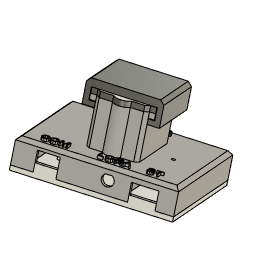
PicoTracker Lora Jig_1.1a v7 (Autodesk Fusion 360 design; units mm, degrees)
Autodesk Fusion 360 part; units mm, degrees
sketch "Sketch1" plane through (0, 0, 0) normal (0, 0, 1) x (1, 0, 0)
  line L0 (-14.5, -3.5) -> (-14.5, 46.5)
  line L1 (-14.5, 46.5) -> (45.5, 46.5)
  line L2 (45.5, 46.5) -> (45.5, -3.5)
  line L3 (-16.5, -5.5) -> (-16.5, 48.5)
  line L4 (-16.5, 48.5) -> (47.5, 48.5)
  line L5 (47.5, 48.5) -> (47.5, -5.5)
  line L6 (-14.5, 46.5) -> (20.5, 46.5)
  line L7 (20.5, 46.5) -> (20.5, 41.5)
  line L8 (20.5, 41.5) -> (-14.5, 41.5)
  line L9 (-14.5, 41.5) -> (-14.5, 46.5)
  line L10 (-14.5, 24.2) -> (20.5, 24.2)
  line L11 (20.5, 24.2) -> (20.5, 21.2)
  line L12 (20.5, 21.2) -> (-14.5, 21.2)
  line L13 (-14.5, 21.2) -> (-14.5, 24.2)
  line L14 (-14.5, 39.5) -> (-16.5, 39.5)
  line L15 (-14.5, 26.2) -> (-16.5, 26.2)
  line L16 (29.5, 46.5) -> (33.5, 46.5)
  line L17 (33.5, 46.5) -> (33.5, 39.5)
  line L18 (33.5, 39.5) -> (29.5, 39.5)
  line L19 (29.5, 39.5) -> (29.5, 46.5)
  line L20 (29.5, 21.2) -> (33.5, 21.2)
  line L21 (33.5, 21.2) -> (33.5, 26.2)
  line L22 (33.5, 26.2) -> (29.5, 26.2)
  line L23 (29.5, 26.2) -> (29.5, 21.2)
  line L24 (20.5, 41.5) -> (20.5, 24.2)
  circle A0 centre (14.5, 32.85) radius 1
  line L25 (-14.5, 1.5) -> (-14.5, -3.5)
  line L26 (45.5, 1.5) -> (45.5, -3.5)
  line L27 (45.5, 46.5) -> (40.5, 46.5)
  line L28 (40.5, 46.5) -> (40.5, 41.5)
  line L29 (40.5, 41.5) -> (45.5, 41.5)
  line L30 (45.5, 41.5) -> (45.5, 46.5)
  circle A1 centre (43, 44) radius 0.9
  circle A2 centre (43, -26) radius 0.9
  circle A3 centre (-12, -26) radius 0.9
  circle A4 centre (-12, 44) radius 0.9
  line L31 (30.5, 0) -> (-1, 0)
  line L32 (-1, 0) -> (-1, 20.5)
  line L33 (-1, 20.5) -> (30.5, 20.5)
  line L34 (30.5, 20.5) -> (30.5, 0)
  arc A5 (-1, 12.75) -> (-1, 7.75) centre (-1, 10.25) ccw
  arc A6 (-1, 15.25) -> (-1, 5.25) centre (-1, 10.25) ccw
  line L35 (-3.5, -2.5) -> (-3.5, 23)
  line L36 (-3.5, 23) -> (33, 23)
  line L37 (33, 23) -> (33, -2.5)
  line L38 (33, -2.5) -> (-3.5, -2.5)
  circle A7 centre (29.1, 10.1) radius 0.85
  circle A8 centre (27.945, 2.48) radius 0.85
  circle A9 centre (25.405, 2.48) radius 0.85
  circle A10 centre (22.865, 2.48) radius 0.85
  circle A11 centre (20.325, 2.48) radius 0.85
  circle A12 centre (17.785, 2.48) radius 0.85
  circle A13 centre (15.245, 2.48) radius 0.85
  circle A14 centre (1.1, 10.1) radius 0.85
  circle A15 centre (1.1, 7.05) radius 0.85
  circle A16 centre (1.1, 13.3) radius 0.85
  circle A17 centre (1.1, 17.1) radius 0.85
  line L39 (26.5, 20.5) -> (3, 20.5)
  line L40 (3, 20.5) -> (3, 4)
  line L41 (26.5, 4) -> (26.5, 20.5)
  line L42 (26.5, 4) -> (3, 4)
  line L43 (14.75, 20.5) -> (14.75, 0)
  circle A18 centre (12.705, 2.48) radius 0.85
  circle A19 centre (10.165, 2.48) radius 0.85
  circle A20 centre (7.625, 2.48) radius 0.85
  circle A21 centre (5.085, 2.48) radius 0.85
  line L44 (-16.5, -5.5) -> (-16.5, -30.5)
  line L45 (-16.5, -30.5) -> (47.5, -30.5)
  line L46 (47.5, -30.5) -> (47.5, -5.5)
  line L47 (-14.5, -7.5) -> (-14.5, -28.5)
  line L48 (-14.5, -28.5) -> (45.5, -28.5)
  line L49 (45.5, -28.5) -> (45.5, -7.5)
  line L50 (45.5, -7.5) -> (45.5, -3.5)
  line L51 (-14.5, -7.5) -> (-14.5, -3.5)
  line L52 (45.5, -28.5) -> (40.5, -28.5)
  line L53 (40.5, -28.5) -> (40.5, -23.5)
  line L54 (40.5, -23.5) -> (45.5, -23.5)
  line L55 (45.5, -23.5) -> (45.5, -28.5)
  line L56 (-14.5, -28.5) -> (22.5, -28.5)
  line L57 (22.5, -28.5) -> (22.5, -23.5)
  line L58 (22.5, -23.5) -> (-14.5, -23.5)
  line L59 (-14.5, -23.5) -> (-14.5, -28.5)
  line L60 (-14.5, -23.5) -> (22.5, -23.5)
  line L61 (22.5, -23.5) -> (22.5, -4.5)
  line L62 (22.5, -4.5) -> (-14.5, -4.5)
  line L63 (-14.5, -4.5) -> (-14.5, -23.5)
  line L64 (-14.5, -4.5) -> (22.5, -4.5)
  line L65 (22.5, -4.5) -> (22.5, -0.5)
  line L66 (22.5, -0.5) -> (-14.5, -0.5)
  line L67 (-14.5, -0.5) -> (-14.5, -4.5)
  line L68 (22.5, -0.5) -> (25.5, -0.5)
  line L69 (25.5, -0.5) -> (25.5, -5.5)
  line L70 (25.5, -5.5) -> (22.5, -5.5)
  line L71 (22.5, -5.5) -> (22.5, -0.5)
  line L72 (22.5, -28.5) -> (25.5, -28.5)
  line L73 (25.5, -28.5) -> (25.5, -22.5)
  line L74 (25.5, -22.5) -> (22.5, -22.5)
  line L75 (22.5, -22.5) -> (22.5, -28.5)
  line L76 (-14.5, -8.5) -> (-16.5, -8.5)
  line L77 (-16.5, -8.5) -> (-16.5, -19.5)
  line L78 (-16.5, -19.5) -> (-14.5, -19.5)
  line L79 (-14.5, -19.5) -> (-14.5, -8.5)
  line L80 (45.5, -23.5) -> (31.5, -23.5)
  line L81 (31.5, -23.5) -> (31.5, 4.5)
  line L82 (31.5, 4.5) -> (45.5, 4.5)
  line L83 (45.5, 4.5) -> (45.5, -23.5)
  line L84 (31.5, -23.5) -> (40.5, -23.5)
  line L85 (40.5, -23.5) -> (40.5, -25.5)
  line L86 (40.5, -25.5) -> (31.5, -25.5)
  line L87 (31.5, -25.5) -> (31.5, -23.5)
  line L88 (31.5, -25.5) -> (29.5, -25.5)
  line L89 (29.5, -25.5) -> (29.5, 4.5)
  line L90 (29.5, 4.5) -> (31.5, 4.5)
  line L91 (31.5, 4.5) -> (31.5, -25.5)
  line L92 (29.5, 4.5) -> (45.5, 4.5)
  line L93 (45.5, 4.5) -> (45.5, 6.5)
  line L94 (45.5, 6.5) -> (29.5, 6.5)
  line L95 (29.5, 6.5) -> (29.5, 4.5)
  line L96 (43.73, 20.7064) -> (43.73, 8.6683) construction
  line L97 (43.73, 8.6683) -> (37.73, 8.6683) construction
  line L98 (37.73, 8.6683) -> (37.73, 20.7064) construction
  line L99 (37.73, 20.7064) -> (43.73, 20.7064) construction
  line L100 (-13.1444, 7.1353) -> (-13.1444, 23.0435) construction
  line L101 (-13.1444, 23.0435) -> (-7.1444, 23.0435) construction
  line L102 (-7.1444, 23.0435) -> (-7.1444, 7.1353) construction
  line L103 (-7.1444, 7.1353) -> (-13.1444, 7.1353) construction
  line L104 (-12.6264, 30.3408) -> (-12.6264, 37.6182) construction
  line L105 (-12.6264, 37.6182) -> (-6.6264, 37.6182) construction
  line L106 (-6.6264, 37.6182) -> (-6.6264, 30.3408) construction
  line L107 (-6.6264, 30.3408) -> (-12.6264, 30.3408) construction
  line L108 (-13.0408, -20.7321) -> (-13.0408, -7.487) construction
  line L109 (-13.0408, -7.487) -> (-7.0408, -7.487) construction
  line L110 (-7.0408, -7.487) -> (-7.0408, -20.7321) construction
  line L111 (-7.0408, -20.7321) -> (-13.0408, -20.7321) construction
  dimension "d57" = 35
  dimension "d58" = 5
  dimension "d59" = 35
  dimension "d60" = 3
  dimension "d61" = 17.3
  dimension "d63" = 2
  dimension "d64" = 7
  dimension "d65" = 4
  dimension "d66" = 4
  dimension "d67" = 5
  dimension "d68" = 9
  dimension "d69" = 9
  dimension "d85" = 2
  dimension "d86" = 8.65
  dimension "d87" = 6
  dimension "d90" = 5
  dimension "d94" = 5
  dimension "d95" = 5
  dimension "d96" = 1.8
  dimension "d97" = 1.8
  dimension "d98" = 1.8
  dimension "d99" = 1.8
  dimension "d144" = 31.5
  dimension "d145" = 20.5
  dimension "d146" = 15
  dimension "d149" = 10.25
  dimension "d150" = 2.5
  dimension "d151" = -2.5
  dimension "d152" = 2.5
  dimension "d153" = 1.7
  dimension "d154" = 1.4
  dimension "d155" = 10.4
  dimension "d156" = 1.7
  dimension "d157" = 2.48
  dimension "d158" = 2.555
  dimension "d161" = -12.7
  dimension "d162" = 0
  dimension "d163" = 1.7
  dimension "d164" = 1.7
  dimension "d165" = 1.7
  dimension "d166" = 1.7
  dimension "d167" = 2.1
  dimension "d168" = 2.1
  dimension "d169" = 2.1
  dimension "d170" = 2.1
  dimension "d171" = 3.4
  dimension "d172" = 7.2
  dimension "d173" = 10.4
  dimension "d174" = 13.45
  dimension "d175" = 4
  dimension "d177" = 4
  dimension "d179" = 4
  dimension "d200" = -10.16
  dimension "d201" = 0
  dimension "d202" = 2.5
  dimension "d203" = 2.5
  dimension "d206" = 75
  dimension "d207" = 5
  dimension "d208" = 5
  dimension "d209" = 2.5
  dimension "d210" = 2.5
  dimension "d211" = 2.5
  dimension "d212" = 2.5
  dimension "d213" = 37
  dimension "d214" = 5
  dimension "d215" = 19
  dimension "d216" = 4
  dimension "d217" = 3
  dimension "d218" = 5
  dimension "d219" = 3
  dimension "d220" = 6
  dimension "d223" = 11
  dimension "d224" = 2
  dimension "d225" = 4
  dimension "d226" = 14
  dimension "d227" = 28
  dimension "d228" = 2
  dimension "d229" = 2
  dimension "d230" = 2
  text T0 "GPS" font "Arial" height 6 align ink ink in box 0 x 0 at (43.73, 20.7064) x (0, -1) y (-1, 0) spacing 1 kerned height is em
  text T1 "LORA" font "Arial" height 6 align ink ink in box 0 x 0 at (-13.1444, 7.1353) x (0, 1) y (1, 0) spacing 1 kerned height is em
  text T2 "ST" font "Arial" height 6 align ink ink in box 0 x 0 at (-12.6264, 30.3408) x (0, 1) y (1, 0) spacing 1 kerned height is em
  text T3 "COM" font "Arial" height 6 align ink ink in box 0 x 0 at (-13.0408, -20.7321) x (0, 1) y (1, 0) spacing 1 kerned height is em
  constraint vertical L0
  constraint horizontal L1
  constraint vertical L2
  constraint horizontal L6
  constraint vertical L7
  constraint horizontal L8
  constraint vertical L9
  constraint horizontal L10
  constraint vertical L11
  constraint horizontal L12
  constraint vertical L13
  constraint coincident L0 L10.start
  constraint coincident L0 L14.start
  constraint coincident L3 L14.end
  constraint perpendicular L3 L14
  constraint coincident L0 L15.start
  constraint coincident L3 L15.end
  constraint perpendicular L3 L15
  constraint horizontal L16
  constraint vertical L17
  constraint horizontal L18
  constraint vertical L19
  constraint coincident L1 L16.start
  constraint horizontal L20
  constraint vertical L21
  constraint horizontal L22
  constraint vertical L23
  constraint collinear L12 L20
  constraint vertical L25
  constraint vertical L26
  constraint horizontal L27
  constraint vertical L28
  constraint horizontal L29
  constraint vertical L30
  constraint horizontal L31
  constraint vertical L32
  constraint horizontal L33
  constraint vertical L34
  constraint coincident L32 A5.centre
  constraint coincident L32 A5.end
  constraint coincident L32 A5.start
  constraint horizontal L39
  constraint vertical L40
  constraint vertical L41
  constraint coincident L33 L39.start
  constraint perpendicular L40 L42
  constraint midpoint L33 L43.start
  constraint midpoint L31 L43.end
  constraint parallel L0 L3
  constraint parallel L1 L4
  constraint parallel L2 L5
  constraint parallel L44 L47
  constraint parallel L45 L48
  constraint parallel L46 L49
  constraint horizontal L76
  constraint vertical L77
  constraint horizontal L78
  constraint vertical L79
  constraint coincident L47 L76.start
  constraint perpendicular L96 L97
  constraint parallel L96 L98
  constraint parallel L97 L99
  constraint perpendicular L100 L101
  constraint parallel L100 L102
  constraint parallel L101 L103
  constraint perpendicular L104 L105
  constraint parallel L104 L106
  constraint parallel L105 L107
  constraint perpendicular L108 L109
  constraint parallel L108 L110
  constraint parallel L109 L111
  measures "d57" distance of L0.end L6.end
  measures "d58" distance of L0.end L8.end
  measures "d59" distance of L10.start L10.end
  measures "d60" distance of L10.start L12.end
  measures "d61" distance of L8 L10
  measures "d63" distance of L10 L15.end
  measures "d64" distance of L16.start L18.end
  measures "d65" distance of L16.start L16.end
  measures "d66" distance of L20.start L20.end
  measures "d67" distance of L20.start L22.end
  measures "d68" distance of L7.end L19
  measures "d69" distance of L11 L23
  measures "d85" diameter of A0
  measures "d86" distance of L8 A0.centre
  measures "d87" distance of L24 A0.centre
  measures "d90" distance of L0.start L25.start
  measures "d94" distance of L1.end L27.end
  measures "d95" distance of L1.end L29.end
  measures "d96" diameter of A1
  measures "d97" diameter of A2
  measures "d98" diameter of A3
  measures "d99" diameter of A4
  measures "d144" distance of L31.start L31.end
  measures "d145" distance of L31.start L33.end
  measures "d146" distance of L2 L34
  measures "d149" distance of L33 A5.centre
  measures "d150" distance of A5
  measures "d152" radius of A5
  measures "d153" diameter of A7
  measures "d154" distance of L34 A7.centre
  measures "d155" distance of L33 A7.centre
  measures "d156" diameter of A8
  measures "d157" distance of L31 A8.centre
  measures "d158" distance of L34 A8.centre
  measures "d163" diameter of A14
  measures "d164" diameter of A15
  measures "d165" diameter of A16
  measures "d166" diameter of A17
  measures "d167" distance of L32 A17.centre
  measures "d168" distance of L32 A16.centre
  measures "d169" distance of L32 A14.centre
  measures "d170" horizontal distance of A5.end A15.centre
  measures "d171" distance of L33 A17.centre
  measures "d172" distance of L33 A16.centre
  measures "d173" distance of L33 A14.centre
  measures "d174" distance of L33 A15.centre
  measures "d175" distance of L34 L41
  measures "d177" distance of L32 L40
  measures "d179" distance of L31 L42
  measures "d202" distance of L1 A4.centre
  measures "d203" distance of L1 A1.centre
  measures "d206" distance of L1 L48
  measures "d207" distance of L48.end L52.end
  measures "d208" distance of L48.end L54.end
  measures "d209" distance of A3.centre L47
  measures "d210" distance of A3.centre L48
  measures "d211" distance of A2.centre L49
  measures "d212" distance of A2.centre L48
  measures "d213" distance of L47.end L56.end
  measures "d214" distance of L47.end L58.end
  measures "d215" distance of L58.end L62.end
  measures "d216" distance of L62.end L66.end
  measures "d217" distance of L65.end L68.end
  measures "d218" distance of L65.end L70.end
  measures "d219" distance of L56.end L72.end
  measures "d220" distance of L56.end L74.end
  measures "d223" distance of L76.start L78.end
  measures "d224" distance of L76.start L76.end
  measures "d225" distance of L62 L76
  measures "d226" distance of L54.end L80.end
  measures "d227" distance of L54.end L82.end
  measures "d228" distance of L80.end L86.end
  measures "d229" distance of L86.end L88.end
  measures "d230" distance of L89.end L94.end
extrude "Extrude5" add sketch "Sketch1" along normal blind 2.5 contours L0 L3 L13 L15 L25 L44 L47 L51 L63 L67 L76 | L0 L25 L35 L38 L51 L62 L64 L65 L66 L67 L71 | L0 L12 L25 A6 L35 L66 | L47 L51 L58 L60 L61 L62 L63 L64 L71 L75 L79 | L35 L38 L65 L66 L71 | L31 L32 A6 L35 L38 L66 L68 L69 L89 | L38 L61 L65 L69 L70 L71 | L0 L10 L11 L12 L13 L35 L36 | L32 A5 A6 L35 | A6 L35 | L38 L65 L68 L69 L71 | L44 L47 L63 L76 L77 L78 L79 | L38 L48 L53 L61 L69 L70 L73 L74 L86 L88 L89 | L0 L8 L10 L24 | L11 L12 L35 L36 | L11 L12 L20 L23 L32 L33 L34 A6 L35 L36 L37 L39 L94 | L32 A5 A6 L35 | L31 L32 L33 A13 L40 L42 L43 | L32 A5 | L0 L1 L2 L3 L4 L5 L6 L9 L14 L16 L26 L27 L30 L44 L45 L46 L47 L48 L49 L50 L52 L55 L56 L59 L63 L72 L78 L83 L93 | L48 L57 L61 L72 L73 L74 L75 | L0 L3 L14 L15 | L1 L2 L7 L11 L17 L18 L19 L20 L21 L22 L23 L24 L28 L29 L36 L37 L94 | L47 L48 L56 L57 L58 L59 L60 L75 | L31 L34 L38 L81 L89 L90 L91 L92 | L38 L81 L87 L88 L89 L91 | L0 L1 L6 L7 L8 L9 | L31 L33 L34 A13 L41 L42 L43 L89 L94 L95 | L37 L38 L81 L82 L91 L92 | L2 L26 L37 L38 L49 L50 L54 L80 L81 L82 L83 L84 L91 L92 | L31 L34 L89 L90 L92 | L20 L23 L36 L37 | L20 L21 L22 L23 L36 L37 | L33 L39 L40 L42 L43 | A13 L43 | L48 L49 L52 L53 L54 L55 L80 L85 | L53 L80 L84 L85 L86 L87 L91 | L34 L37 L82 L90 L92 L94 | L34 L90 L92 L94 L95 | L1 L16 L17 L18 L19 | L33 L39 L41 L42 L43 | L2 L37 L82 L92 L93 L94 | L1 L2 L27 L28 L29 L30 | A1 | A2 | A3 | A4 picked at (14.6679, 2.3414) makes body 1
extrude "Extrude6" add sketch "Sketch1" against normal blind 10 contours L31 L32 L33 A13 L40 L42 L43 | L32 A5 | L31 L33 L34 A13 L41 L42 L43 L89 L94 L95 | L31 L34 L89 L90 L92 | L34 L90 L92 L94 L95 bodies 1
extrude "Extrude7" add sketch "Sketch1" against normal blind 17 contours L33 L39 L40 L42 L43 | L33 L39 L41 L42 L43 bodies 1
extrude "Extrude8" add sketch "Sketch1" against normal blind 24 contours L35 L38 L65 L66 L71 | L31 L32 A6 L35 L38 L66 L68 L69 L89 | L32 A5 A6 L35 | A6 L35 | L38 L65 L68 L69 L71 | L11 L12 L35 L36 | L11 L12 L20 L23 L32 L33 L34 A6 L35 L36 L37 L39 L94 | L32 A5 A6 L35 | L31 L34 L38 L81 L89 L90 L91 L92 | L37 L38 L81 L82 L91 L92 | L20 L23 L36 L37 | L34 L37 L82 L90 L92 L94 bodies 1
extrude "Extrude9" add sketch "Sketch1" along normal blind 12.5 contours L0 L25 L35 L38 L51 L62 L64 L65 L66 L67 L71 | L38 L61 L65 L69 L70 L71 | L0 L10 L11 L12 L13 L35 L36 | L11 L12 L35 L36 | L48 L57 L61 L72 L73 L74 L75 | L47 L48 L56 L57 L58 L59 L60 L75 | L38 L81 L87 L88 L89 L91 | L0 L1 L6 L7 L8 L9 | L20 L23 L36 L37 | L20 L21 L22 L23 L36 L37 | L48 L49 L52 L53 L54 L55 L80 L85 | L53 L80 L84 L85 L86 L87 L91 | L1 L16 L17 L18 L19 | L2 L37 L82 L92 L93 L94 | L1 L2 L27 L28 L29 L30 bodies 1
extrude "Extrude10" add sketch "Sketch1" along normal blind 4.5 contours L0 L3 L14 L15 bodies 1
extrude "Extrude25" add sketch "Sketch1" along normal blind 3.5 contours L44 L47 L63 L76 L77 L78 L79 bodies 1
extrude "Extrude13" add sketch "Sketch1" along normal blind 14 contours L0 L3 L13 L15 L25 L44 L47 L51 L63 L67 L76 | L0 L1 L2 L3 L4 L5 L6 L9 L14 L16 L26 L27 L30 L44 L45 L46 L47 L48 L49 L50 L52 L55 L56 L59 L63 L72 L78 L83 L93 bodies 1
extrude "Extrude26" add sketch "Sketch1" against normal blind 1.5 text T3 T1 T2 T0 bodies 1
chamfer "Chamfer1" distance 2 angle 45 8 edges at (15.5, 48.5, 0) (-16.5, 9, 0) (47.5, 9, 0) (33, -2.5, -12) (-3.5, -2.5, -12) (-3.5, 23, -12) (33, 23, -12) (15.5, -30.5, 0) on bodies 1
extrude "Extrude11" add sketch "Sketch1" along normal blind 3.5 contours L0 L8 L10 L24 bodies 1
sketch "Sketch2" plane through (0, 0, -24) normal (0, 0, -1) x (-1, 0, 0)
  line L0 (-30.5, 20.5) -> (1, 20.5)
  line L1 (1, 20.5) -> (1, 12.75)
  arc A0 (1, 7.75) -> (1, 12.75) centre (1, 10.25) ccw
  line L2 (1, 7.75) -> (1, 0)
  line L3 (1, 0) -> (-30.5, 0)
  line L4 (-30.5, 0) -> (-30.5, 20.5)
  arc A1 (3.5, 5.9199) -> (3.5, 14.5801) centre (1, 10.25) ccw
  line L5 (3.5, 14.5801) -> (3.5, 21)
  line L6 (1.5, 23) -> (-31, 23)
  line L7 (-33, 21) -> (-33, -0.5)
  line L8 (-31, -2.5) -> (1.5, -2.5)
  line L9 (3.5, -0.5) -> (3.5, 5.9199)
  line L10 (-31, 23) -> (-33, 21)
  line L11 (-33, -0.5) -> (-31, -2.5)
  line L12 (1.5, -2.5) -> (3.5, -0.5)
  line L13 (3.5, 21) -> (1.5, 23)
  line L14 (-31, 23) -> (1.5083, 23)
  line L15 (1.5083, 23) -> (1.5083, 26)
  line L16 (1.5083, 26) -> (-31, 26)
  line L17 (-31, 26) -> (-31, 23)
  line L18 (-31, -2.5) -> (1.5, -2.5)
  line L19 (1.5, -2.5) -> (1.5, -5.5)
  line L20 (1.5, -5.5) -> (-31, -5.5)
  line L21 (-31, -5.5) -> (-31, -2.5)
  dimension "d180" = 3
  dimension "d181" = 3
  constraint horizontal L14
  constraint vertical L15
  constraint horizontal L16
  constraint vertical L17
  constraint coincident L6.end L10.start
  constraint horizontal L18
  constraint vertical L19
  constraint horizontal L20
  constraint vertical L21
  constraint coincident L8.start L11.end
  measures "d180" distance of L6.end L16.end
  measures "d181" distance of L8.start L20.end
extrude "Extrude12" add sketch "Sketch2" against normal blind 3 contours L8 L18 L19 L20 L21 | L6 L14 L15 L16 L17 bodies 1
extrude "Extrude14" add sketch "Sketch2" along normal blind 3 separate body contours L0 L1 A0 L2 L3 L4 | A1 L5 L6 L7 L8 L9 L10 L11 L12 L13 L14 L18 | L8 L18 L19 L20 L21 | L6 L14 L15 L16 L17 makes body 2
extrude "Extrude15" add sketch "Sketch2" against normal blind 3 contours L0 L1 A0 L2 L3 L4 bodies 2
sketch "Sketch3" plane through (0, 0, 14) normal (0, 0, 1) x (1, 0, 0)
  line L0 (45.5, 46.5) -> (45.5, -28.5)
  line L1 (-14.5, -28.5) -> (-14.5, -19.5)
  line L2 (-16.5, -19.5) -> (-16.5, -30.5)
  line L3 (47.5, -30.5) -> (47.5, 48.5)
  line L4 (47.5, 48.5) -> (-16.5, 48.5)
  line L5 (-16.5, 48.5) -> (-16.5, 39.5)
  line L6 (-16.5, 39.5) -> (-14.5, 39.5)
  line L7 (-14.5, 46.5) -> (45.5, 46.5)
  line L8 (-14.5, 41.5) -> (20.5, 41.5)
  line L9 (20.5, 41.5) -> (20.5, 24.2)
  line L10 (20.5, 24.2) -> (-14.5, 24.2)
  line L11 (-14.5, 24.2) -> (-14.5, 41.5)
  line L12 (-16.5, 39.5) -> (-14.5, 39.5)
  line L13 (-14.5, -19.5) -> (-16.5, -19.5)
  line L14 (-16.5, -19.5) -> (-16.5, 39.5)
  line L15 (-16.5, 48.5) -> (47.5, 48.5)
  line L16 (47.5, 48.5) -> (47.5, -30.5)
  line L17 (47.5, -30.5) -> (-16.5, -30.5)
  line L18 (-16.5, -30.5) -> (-16.5, 48.5)
  circle A0 centre (-12, 44) radius 1.1
  circle A1 centre (43, 44) radius 1.1
  line L19 (-16.5, -30.5) -> (47.5, -30.5)
  line L20 (45.5, -28.5) -> (-14.5, -28.5)
  line L21 (-14.5, -19.5) -> (-16.5, -19.5)
  circle A2 centre (42.9969, -26.0001) radius 1.1
  circle A3 centre (-11.9905, -26.0415) radius 1.1
  line L22 (45.5, -28.5) -> (-14.5, -28.5)
  line L23 (-14.5, -28.5) -> (-14.5, 46.5)
  line L24 (-14.5, 46.5) -> (45.5, 46.5)
  line L25 (45.5, 46.5) -> (45.5, -28.5)
  line L26 (20.5, 41.5) -> (-14.5, 41.5)
  line L27 (-14.5, 26.22) -> (-16.5, 26.22)
  line L28 (-14.5, -8.5082) -> (-16.5, -8.4971)
  line L29 (15.5, -11.5) -> (3.5, -11.5)
  line L30 (3.5, -11.5) -> (3.5, -16.5)
  line L31 (3.5, -16.5) -> (15.5, -16.5)
  line L32 (15.5, -16.5) -> (15.5, -11.5)
  line L33 (22.5, -23.5) -> (-14.5, -23.5)
  line L34 (-14.5, -19.5) -> (-14.5, -8.5)
  line L35 (41.4886, -5.5) -> (35.4886, -5.5)
  line L36 (35.4886, -5.5) -> (35.4886, -13.5)
  line L37 (35.4886, -13.5) -> (41.4886, -13.5)
  line L38 (41.4886, -13.5) -> (41.4886, -5.5)
  line L39 (45.5, -23.5) -> (31.5, -23.5)
  point P0 (20.5, 24.2)
  point P1 (-14.5, 41.5)
  dimension "d110" = 2.2
  dimension "d111" = 2.2
  dimension "d233" = 2.2
  dimension "d234" = 2.2
  dimension "d235" = 2
  dimension "d240" = 12
  dimension "d241" = 5
  dimension "d242" = 7
  dimension "d243" = 18
  dimension "d244" = 6
  dimension "d245" = 8
  dimension "d246" = 10
  constraint horizontal L8
  constraint vertical L9
  constraint horizontal L10
  constraint vertical L11
  constraint coincident P0 L9.end
  constraint horizontal L12
  constraint horizontal L13
  constraint vertical L14
  constraint coincident L1.end L13.start
  constraint coincident L5.end L6.start
  constraint horizontal L15
  constraint vertical L16
  constraint horizontal L17
  constraint vertical L18
  constraint coincident L3.start L16.end
  constraint coincident L4.end L5.start
  constraint coincident P1 L8.start
  constraint perpendicular L11 L26
  constraint coincident L11 L27.start
  constraint coincident L23 L27.start
  constraint coincident L14 L27.end
  constraint perpendicular L14 L27
  constraint coincident L23 L28.start
  constraint coincident L14 L28.end
  constraint horizontal L29
  constraint vertical L30
  constraint horizontal L31
  constraint vertical L32
  constraint horizontal L35
  constraint vertical L36
  constraint horizontal L37
  constraint vertical L38
  measures "d110" diameter of A0
  measures "d111" diameter of A1
  measures "d233" diameter of A2
  measures "d234" diameter of A3
  measures "d240" distance of L29.start L29.end
  measures "d241" distance of L29.start L31.end
  measures "d242" distance of L31 L33
  measures "d243" distance of L30 L34
  measures "d244" distance of L35.start L35.end
  measures "d245" distance of L35.start L37.end
  measures "d246" distance of L37 L39
extrude "Extrude16" add sketch "Sketch3" against normal blind 1.5 separate body contours L0 L1 L7 L8 L9 L10 L20 L22 L23 L24 L25 L26 L34 | L29 L30 L31 L32 | L35 L36 L37 L38 makes body 3
extrude "Extrude17" add sketch "Sketch3" against normal blind 2.5 contours L8 L9 L10 L11 L23 L26 bodies 3
extrude "Extrude18" add sketch "Sketch3" along normal blind 2.5 contours L0 L1 L2 L3 L4 L5 L6 L7 L11 L12 L13 L15 L16 L17 L18 L19 L20 L21 L22 L23 L24 L25 | L0 L1 L7 L8 L9 L10 L20 L22 L23 L24 L25 L26 L34 | L8 L9 L10 L11 L23 L26 | L6 L11 L12 L14 L18 L23 L27 | L11 L14 L18 L23 L27 L28 L34 | L13 L14 L18 L21 L23 L28 L34 | L29 L30 L31 L32 | L35 L36 L37 L38 bodies 3
extrude "Extrude19" add sketch "Sketch3" against normal blind 3.5 contours L6 L11 L12 L14 L18 L23 L27 bodies 3
extrude "Extrude27" add sketch "Sketch3" against normal blind 4.5 contours L13 L14 L18 L21 L23 L28 L34 bodies 3
extrude "Extrude28" add sketch "Sketch3" against normal blind 8 contours L29 L30 L31 L32 | L35 L36 L37 L38 bodies 3
chamfer "Chamfer2" distance 1.5 angle 45 4 edges at (-13.016, -25.6438, 16.5) (41.9714, -25.6023, 16.5) (41.9744, 44.3978, 16.5) (-13.0256, 44.3978, 16.5) on bodies 3
sketch "Sketch4" plane through (-3.5, 0, 0) normal (-1, 0, 0) x (0, 0, 1)
  line L0 (-31, 19) -> (-31, -5.5)
  line L1 (-31, -5.5) -> (-27, -5.5)
  line L2 (-21, -2.5) -> (-18, -2.5)
  line L3 (-18, -2.5) -> (-18, -5.5)
  line L4 (-18, -5.5) -> (-21, -5.5)
  line L5 (-21, -5.5) -> (-21, -2.5)
  line L6 (-18, 29) -> (-31, 29)
  line L7 (-31, 29) -> (-31, 19)
  line L8 (-31, -5.5) -> (-18, -5.5)
  line L9 (-18, -5.5) -> (-18, -8.5)
  line L10 (-18, -8.5) -> (-31, -8.5)
  line L11 (-31, -8.5) -> (-31, -5.5)
  line L12 (-21, -2.5) -> (-20.7, -2.5)
  line L13 (-20.7, -2.5) -> (-20.7, -5.5)
  line L14 (-20.7, -5.5) -> (-21, -5.5)
  line L15 (-21, -5.5) -> (-21, -2.5)
  line L16 (-27, -5.5) -> (-20.7026, -5.5)
  line L17 (-20.7026, -5.5) -> (-20.7026, -5.7)
  line L18 (-20.7026, -5.7) -> (-27, -5.7)
  line L19 (-27, -5.7) -> (-27, -5.5)
  line L20 (-27, 26.2) -> (-20.7, 26.2)
  line L21 (-20.7, 26.2) -> (-20.7, 23)
  line L22 (-18, 29) -> (-18, 23.0003)
  line L23 (-18, 23.0003) -> (-20.7, 23)
  line L24 (-27, 26.2) -> (-27, 26)
  line L25 (-27, 26.2) -> (-27, -5.5)
  line L26 (0, 46.5) -> (0, -28.5)
  dimension "d124" = 3
  dimension "d125" = 3
  dimension "d126" = 3
  dimension "d129" = 0.3
  dimension "d130" = 0.2
  dimension "d183" = 6.3
  dimension "d185" = 3.2
  dimension "d197" = 27
  constraint vertical L0
  constraint horizontal L1
  constraint horizontal L2
  constraint vertical L3
  constraint horizontal L4
  constraint vertical L5
  constraint horizontal L6
  constraint vertical L7
  constraint horizontal L8
  constraint vertical L9
  constraint horizontal L10
  constraint vertical L11
  constraint horizontal L12
  constraint vertical L13
  constraint horizontal L14
  constraint vertical L15
  constraint horizontal L16
  constraint vertical L17
  constraint horizontal L18
  constraint vertical L19
  constraint perpendicular L20 L21
  constraint perpendicular L6 L22
  constraint perpendicular L8 L25
  measures "d124" distance of L2.start L4.end
  measures "d125" distance of L2.start L2.end
  measures "d126" distance of L0.end L10.end
  measures "d129" distance of L2.start L12.end
  measures "d130" distance of L1.end L18.end
  measures "d183" distance of L20.start L20.end
  measures "d185" distance of L20.end L21.end
  measures "d197" distance of L25 L26
extrude "Extrude20" add sketch "Sketch4" against normal blind 32.5 from surface at -2 separate body contours L0 L1 L6 L7 L8 L20 L21 L22 L23 L24 L25 | L1 L4 L8 L9 L10 L11 L14 L17 L18 L19 | L2 L3 L4 L8 L13 makes body 4
chamfer "Chamfer3" distance 2 angle 45 2 edges at (14.75, 29, -31) (14.75, -8.5, -31) on bodies 4
sketch "Sketch5" plane through (-14.5, 0, 0) normal (1, 0, 0) x (0, 0, -1)
  line L0 (-14, 46.5) -> (-14, 39.5)
  line L1 (-14, 39.5) -> (-4.5, 39.5)
  line L2 (-4.5, 39.5) -> (-4.5, 26.2)
  line L3 (-4.5, 26.2) -> (-14, 26.2)
  circle A0 centre (-7, 15.2) radius 3.1
  line L4 (-2.8, 17.6249) -> (-7, 20.0497)
  line L5 (-7, 20.0497) -> (-11.2, 17.6249)
  line L6 (-11.2, 17.6249) -> (-11.2, 12.7751)
  line L7 (-11.2, 12.7751) -> (-7, 10.3503)
  line L8 (-7, 10.3503) -> (-2.8, 12.7751)
  line L9 (-2.8, 12.7751) -> (-2.8, 17.6249)
  line L10 (-2.5, 19.1686) -> (-2.5, 11.2314)
  arc A1 (-2.5, 19.1686) -> (-2.5, 11.2314) centre (-7, 15.2) ccw
  line L11 (-4.3829, 16.8616) -> (-4.3829, 13.5384)
  line L12 (-12.5, 17.5979) -> (-12.5, 12.8021)
  line L13 (-3.5, 24.2) -> (-3.5, 41.5)
  line L14 (-3.5, 41.5) -> (-12.5, 41.5)
  line L15 (-12.5, 41.5) -> (-12.5, 46.5)
  line L16 (-12.5, 46.5) -> (-14, 46.5)
  line L17 (-14, 26.2) -> (-14, -8.5)
  line L18 (-14, -8.5) -> (-3.5, -8.5)
  line L19 (-3.5, -8.5) -> (-3.5, -19.5)
  line L20 (-3.5, -19.5) -> (-14, -19.5)
  line L21 (-14, -19.5) -> (-14, -28.5)
  line L22 (-14, -28.5) -> (-12.5, -28.5)
  line L23 (-12.5, -28.5) -> (-12.5, -23.5)
  line L24 (-12.5, -23.5) -> (-2.5, -23.5)
  line L25 (-2.5, -23.5) -> (-2.5, -4.5)
  line L26 (-2.5, -4.5) -> (-12.5, -4.5)
  line L27 (-12.5, -4.5) -> (-12.5, -0.5)
  line L28 (-12.5, -0.5) -> (-2.5, -0.5)
  line L29 (-2.5, -0.5) -> (-2.5, 21.2)
  line L30 (-2.5, 21.2) -> (-12.5, 21.2)
  line L31 (-12.5, 21.2) -> (-12.5, 24.2)
  line L32 (-12.5, 24.2) -> (-3.5, 24.2)
  point P0 (-7, 15.2)
  dimension "d135" = 6.2
  dimension "d137" = 4.2
  dimension "d139" = 12
  constraint coincident P0 A0.centre
  constraint concentric A0 A1
  constraint coincident A0 L11.start
  constraint coincident A0 L11.end
  constraint vertical L11
  constraint coincident A1 L12.start
  constraint coincident A1 L12.end
  measures "d135" diameter of A0
  measures "d137" distance of P0 L9
  measures "d139" diameter of A1
extrude "Extrude21" add sketch "Sketch5" along normal blind 2 contours L10 A1 L12 L29 bodies 1
extrude "Extrude22" cut sketch "Sketch5" against normal blind 2 contours A0 L11 picked at (-7.2749, 14.9188) bodies 1
sketch "Sketch6" plane through (47.5, 0, 0) normal (1, 0, 0) x (0, 0, -1)
  line L0 (-2, -30.5) -> (-2, 48.5)
  line L1 (-2, 48.5) -> (-14, 48.5)
  circle A0 centre (-7.0046, 15.1824) radius 3.125
  line L2 (-6.9782, 20.0321) -> (-11.1913, 17.63)
  line L3 (-11.1913, 17.63) -> (-11.2177, 12.7804)
  line L4 (-11.2177, 12.7804) -> (-7.0309, 10.3327)
  line L5 (-7.0309, 10.3327) -> (-2.8178, 12.7347)
  line L6 (-2.8178, 12.7347) -> (-2.7915, 17.5844)
  line L7 (-2.7915, 17.5844) -> (-6.9782, 20.0321)
  line L8 (-2.4792, 19.1221) -> (-2.5223, 11.1938)
  arc A1 (-2.4792, 19.1221) -> (-2.5223, 11.1938) centre (-7.0046, 15.1824) ccw
  line L9 (-4.3828, 16.883) -> (-4.3828, 13.4818)
  line L10 (-14, -30.5) -> (-2, -30.5)
  line L11 (-14, 48.5) -> (-14, -30.5)
  point P0 (-7.0046, 15.1824)
  dimension "d187" = 6.25
  dimension "d188" = 12
  dimension "d189" = 8.4
  constraint coincident P0 A0.centre
  constraint parallel L6 L8
  constraint coincident A0 L9.start
  constraint coincident A0 L9.end
  constraint vertical L9
  measures "d187" diameter of A0
  measures "d188" diameter of A1
  measures "d189" distance of L4 L7
extrude "Extrude23" add sketch "Sketch6" against normal blind 2 from surface at -2 contours L8 A1 bodies 1
extrude "Extrude24" cut sketch "Sketch6" against normal blind 2 contours A0 L9 picked at (-6.2292, 14.809) bodies 1
named bodies: "LoRa Jig Body", "LoRa Jig Top Cap", "LoRa Jig  Bottom", "LoRa Jig Clip"
